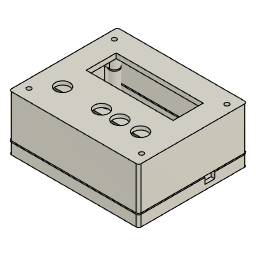
hotplate controller case v5 (Autodesk Fusion 360 design; units mm, degrees)
Autodesk Fusion 360 part; units mm, degrees
note: some values were not read from the file. Set by a fixed rule: which sketch regions a step uses.
sketch "Sketch1" plane through (0, 0, 0) normal (0, 0, 1) x (1, 0, 0)
  line L0 (0.5, 79.5) -> (106.9, 79.5)
  line L1 (106.9, 79.5) -> (106.9, -9.5)
  line L2 (106.9, -9.5) -> (0.5, -9.5)
  line L3 (0.5, -9.5) -> (0.5, 79.5)
  circle A0 centre (-121.3001, 1.3) radius 5
  line L4 (-51.3001, 1.3) -> (-121.3001, 1.3) construction
  line L5 (-139.5001, 79.5) -> (-33.1001, 79.5)
  circle A1 centre (-121.3001, 68.7) radius 1.8
  line L6 (-139.5001, -9.5) -> (-139.5001, 79.5)
  line L7 (-33.1001, 79.5) -> (-33.1001, -9.5)
  circle A2 centre (-51.3001, 1.3) radius 5
  line L8 (-51.3001, 68.7) -> (-51.3001, 1.3) construction
  line L9 (-121.3001, 1.3) -> (-121.3001, 68.7) construction
  circle A3 centre (-121.3001, 68.7) radius 5
  circle A4 centre (-51.3001, 1.3) radius 1.8
  circle A5 centre (-121.3001, 1.3) radius 1.8
  line L10 (-121.3001, 68.7) -> (-51.3001, 68.7) construction
  circle A6 centre (-51.3001, 68.7) radius 1.8
  line L11 (-136.5, 76.5) -> (-36.1001, 76.5)
  line L12 (-33.1001, -9.5) -> (-139.5001, -9.5)
  circle A7 centre (-51.3001, 68.7) radius 5
  circle A8 centre (-130, 62) radius 1.8
  circle A9 centre (-42, 62) radius 1.8
  circle A10 centre (-130, 8) radius 1.8
  circle A11 centre (-42, 8) radius 1.8
  circle A12 centre (-132.5001, 0) radius 1.8
  circle A13 centre (-132.5001, 70) radius 1.8
  circle A14 centre (-40.1001, 70) radius 1.8
  circle A15 centre (-40.1001, 0) radius 1.8
  line L13 (-136.5, 74) -> (-136.5, 76.5)
  line L14 (-132.5001, 74) -> (-136.5, 74)
  line L15 (-38.6001, 74) -> (-36.1001, 74)
  circle A16 centre (7.4999, 70) radius 1.8
  circle A17 centre (99.8999, 70) radius 1.8
  circle A18 centre (7.4999, 0) radius 1.8
  circle A19 centre (99.8999, 0) radius 1.8
  line L16 (-36.1001, 66) -> (-36.1001, 4)
  line L17 (-36.1001, -6.5) -> (-136.5001, -6.5)
  line L18 (-132.5001, 4) -> (-136.5, 4)
  line L19 (-134.0029, 66) -> (-136.5001, 66)
  line L20 (-36.1001, 76.5) -> (-36.1001, 74)
  line L21 (-40.0992, 66) -> (-36.1001, 66)
  line L22 (-38.6001, 4) -> (-36.1001, 4)
  line L23 (-36.1001, -4) -> (-40.0992, -4)
  line L24 (-36.1001, -4) -> (-36.1001, -6.5)
  line L25 (-134.0029, -4) -> (-136.5001, -4)
  line L26 (-136.5001, -4) -> (-136.5001, -6.5)
  line L27 (-136.5001, 66) -> (-136.5, 4)
  line L28 (-136.5, 15) -> (-139.5001, 15)
  line L29 (-136.5, 23) -> (-139.5001, 23)
  line L30 (-136.5, 45) -> (-139.5001, 45)
  line L31 (-136.5, 53) -> (-139.5001, 53)
  line L32 (7.4999, 4) -> (3.5, 4)
  arc A20 (7.4971, -4) -> (7.4999, 4) centre (7.4999, 0) ccw
  line L33 (7.4971, -4) -> (3.4999, -4)
  line L34 (3.4999, -4) -> (3.4999, -6.5)
  line L35 (103.8999, -6.5) -> (3.4999, -6.5)
  line L36 (103.8999, -4) -> (103.8999, -6.5)
  line L37 (103.8999, -4) -> (99.9008, -4)
  arc A21 (99.8999, 4) -> (99.9008, -4) centre (99.8999, 0) ccw
  line L38 (99.8999, 4) -> (103.8999, 4)
  line L39 (103.8999, 66) -> (103.8999, 4)
  line L40 (99.9008, 66) -> (103.8999, 66)
  arc A22 (99.8999, 74) -> (99.9008, 66) centre (99.8999, 70) ccw
  line L41 (99.8999, 74) -> (103.8999, 74)
  line L42 (103.8999, 76.5) -> (103.8999, 74)
  line L43 (3.5, 76.5) -> (103.8999, 76.5)
  line L44 (3.5, 74) -> (3.5, 76.5)
  line L45 (7.4999, 74) -> (3.5, 74)
  arc A23 (7.4971, 66) -> (7.4999, 74) centre (7.4999, 70) ccw
  line L46 (7.4971, 66) -> (3.4999, 66)
  line L47 (3.4999, 66) -> (3.5, 4)
  circle A24 centre (-132.5001, 0) radius 4
  circle A25 centre (-132.5001, 70) radius 4
  circle A26 centre (-40.1001, 0) radius 4
  circle A27 centre (-40.1001, 70) radius 4
  line L48 (-38.6001, 74) -> (-40.1001, 74)
  line L49 (-38.6001, 4) -> (-40.1001, 4)
  line L50 (-134.0029, -4) -> (-132.5001, -4)
  line L51 (-134.0029, 66) -> (-132.5001, 66)
  line L52 (3.5, 4) -> (3.4999, -4)
  line L53 (103.8999, 4) -> (103.8999, -4)
  line L54 (103.8999, 74) -> (103.8999, 66)
  line L55 (3.5, 74) -> (3.4999, 66)
  circle A28 centre (20, 15) radius 5.9
  circle A29 centre (52, 15) radius 5.9
  circle A30 centre (67, 15) radius 5.9
  circle A31 centre (84, 15) radius 5.9
  line L56 (17.9999, 61) -> (89.3999, 61)
  line L57 (89.3999, 61) -> (89.3999, 36.4)
  line L58 (89.3999, 36.4) -> (17.9999, 36.4)
  line L59 (17.9999, 36.4) -> (17.9999, 61)
  line L60 (89.3999, 60) -> (94.3999, 60)
  line L61 (94.3999, 60) -> (94.3999, 37.4)
  line L62 (94.3999, 37.4) -> (89.3999, 37.4)
  line L63 (14, 67) -> (94.3999, 67)
  line L64 (94.3999, 67) -> (94.3999, 31.9055)
  line L65 (94.3999, 31.9055) -> (14, 31.9055)
  line L66 (14, 31.9055) -> (14, 67)
  circle A32 centre (8, 15) radius 1.8
  circle A33 centre (37, 15) radius 1.8
  circle A34 centre (96, 15) radius 1.8
  circle A35 centre (37, 15) radius 4
  line L67 (-33.1001, 53) -> (-36.1001, 53)
  line L68 (-33.1001, 45) -> (-36.1001, 45)
  circle A36 centre (8, 15) radius 4
  circle A37 centre (8, 15) radius 1.8
  circle A38 centre (37, 15) radius 1.8
  circle A39 centre (37, 15) radius 4
  circle A40 centre (96, 15) radius 4
  circle A41 centre (96, 15) radius 1.8
  circle A42 centre (157, 15) radius 1.8
  circle A43 centre (128, 15) radius 1.8
  line L69 (124, 22) -> (124, 8)
  circle A44 centre (187, 15) radius 1
  circle A45 centre (140, 15) radius 1
  circle A46 centre (172, 15) radius 1
  circle A47 centre (157, 15) radius 1.8
  circle A48 centre (216, 15) radius 1.8
  circle A49 centre (204, 15) radius 1
  circle A50 centre (216, 15) radius 1.8
  circle A51 centre (128, 15) radius 1.8
  line L70 (124, 22) -> (220, 22)
  line L71 (220, 22) -> (220, 8)
  line L72 (220, 8) -> (124, 8)
  circle A52 centre (137.9, 11.5) radius 0.75
  circle A53 centre (142.1, 11.5) radius 0.75
  circle A54 centre (174.1, 11.5) radius 0.75
  circle A55 centre (169.9, 11.5) radius 0.75
  circle A56 centre (189.1, 11.5) radius 0.75
  circle A57 centre (184.9, 11.5) radius 0.75
  circle A58 centre (206.1, 11.5) radius 0.75
  circle A59 centre (201.9, 11.5) radius 0.75
  point P0 (-120, 0)
  dimension "d22" = 3.6
  dimension "d23" = 3.6
  dimension "d24" = 3.6
  dimension "d25" = 3.6
  dimension "d30" = 10
  dimension "d31" = 10
  dimension "d32" = 10
  dimension "d43" = 3.6
  dimension "d44" = 3.6
  dimension "d59" = 11.8
  dimension "d60" = 11.8
  dimension "d61" = 11.8
  dimension "d62" = 11.8
  dimension "d68" = 71.4
  dimension "d69" = 5
  dimension "d70" = 24.6
  dimension "d97" = 2
  dimension "d98" = 2
  dimension "d99" = 2
  dimension "d100" = 2
  constraint coincident L8.start L10.end
  constraint coincident L4.start A2.centre
  constraint coincident A1.centre L9.end
  constraint coincident A0.centre L4.end
  constraint concentric A1 A3
  constraint concentric A0 A5
  constraint concentric A2 A4
  constraint concentric A6 A7
  constraint perpendicular L15 L20
  constraint perpendicular L16 L21
  constraint perpendicular L17 L24
  constraint perpendicular L17 L26
  constraint coincident L6 L28.end
  constraint perpendicular L6 L28
  constraint coincident L6 L29.end
  constraint perpendicular L6 L29
  constraint coincident L27 L29.start
  constraint coincident L27 L28.start
  constraint coincident L6 L30.end
  constraint perpendicular L6 L30
  constraint coincident L6 L31.end
  constraint perpendicular L6 L31
  constraint coincident L27 L31.start
  constraint coincident L27 L30.start
  constraint tangent L45 A23
  constraint perpendicular L41 L42
  constraint perpendicular L39 L40
  constraint tangent A21 L38
  constraint perpendicular L35 L36
  constraint perpendicular L34 L35
  constraint coincident L18.start A24
  constraint tangent L18 A24
  constraint concentric A13 A25
  constraint coincident L14.start A25
  constraint tangent L14 A25
  constraint concentric A15 A26
  constraint coincident L23.end A26
  constraint concentric A14 A27
  constraint coincident L21.start A27
  constraint coincident A27 L48.end
  constraint tangent A27 L48
  constraint parallel L15 L48
  constraint coincident A26 L49.end
  constraint tangent A26 L49
  constraint horizontal L49
  constraint coincident A24 L50.end
  constraint tangent A24 L50
  constraint coincident A25 L51.end
  constraint tangent A25 L51
  constraint perpendicular L37 L53
  constraint perpendicular L40 L54
  constraint horizontal L56
  constraint vertical L57
  constraint horizontal L58
  constraint vertical L59
  constraint horizontal L60
  constraint vertical L61
  constraint horizontal L62
  constraint coincident L57 L60.start
  constraint coincident L57 L62.end
  constraint horizontal L63
  constraint vertical L64
  constraint horizontal L65
  constraint vertical L66
  constraint concentric A33 A35
  constraint coincident L7 L67.start
  constraint perpendicular L7 L67
  constraint coincident L7 L68.start
  constraint coincident L16 L67.end
  constraint coincident L16 L68.end
  constraint concentric A36 A37
  constraint concentric A40 A41
  constraint concentric A38 A39
  constraint horizontal L70
  constraint vertical L71
  constraint horizontal L72
  measures "d22" diameter of A6
  measures "d23" diameter of A4
  measures "d24" diameter of A1
  measures "d25" diameter of A5
  measures "d30" diameter of A0
  measures "d31" diameter of A2
  measures "d32" diameter of A7
  measures "d43" diameter of A12
  measures "d44" diameter of A13
  measures "d59" diameter of A28
  measures "d60" diameter of A29
  measures "d61" diameter of A30
  measures "d62" diameter of A31
  measures "d68" distance of L56.start L56.end
  measures "d69" distance of L61.end L62.end
  measures "d70" distance of L56.start L58.end
  measures "d97" diameter of A45
  measures "d98" diameter of A46
  measures "d99" diameter of A44
  measures "d100" diameter of A49
extrude "Extrude1" add sketch "Sketch1" along normal blind 3 contours L11 L13 L14 L15 L16 L17 L18 L19 L20 L21 L22 L23 L24 L25 L26 L27 A24 A25 A26 A27 L48 L49 L50 L51 makes body 1
extrude "Extrude2" add sketch "Sketch1" along normal blind 9 contours L5 L6 L7 L11 L13 L14 L15 L16 L19 L20 L21 L27 L31 A25 A27 L48 L51 L67 | L6 L27 L29 L30 | L6 L7 L12 L16 L17 L18 L22 L23 L24 L25 L26 L27 L28 A24 A26 L49 L50 L68 bodies 1
extrude "Extrude3" add sketch "Sketch1" along normal blind 4 contours L5 L6 L7 L11 L13 L14 L15 L16 L19 L20 L21 L27 L31 A25 A27 L48 L51 L67 | L6 L27 L30 L31 | L7 L16 L67 L68 | L6 L27 L28 L29 bodies 1
extrude "Extrude4" add sketch "Sketch1" along normal blind 7 contours A0 | A2 | A3 | A7 bodies 1
extrude "Extrude6" add sketch "Sketch1" along normal blind 25 contours A27 | A25 | A26 | A24 bodies 1
chamfer "Chamfer1" distance 1.5 angle 45 4 edges at (-131.6782, 62.6509, 3) (-43.6782, 62.6509, 3) (-43.6782, 8.6509, 3) (-131.6782, 8.6509, 3) on bodies 1
extrude "Extrude5" add sketch "Sketch1" against normal blind 35 separate body contours L0 L1 L2 L3 makes body 2
extrude "Extrude7" add sketch "Sketch1" against normal blind 3 contours L32 A20 L33 L34 L35 L36 L37 A21 L38 L39 L40 A22 L41 L42 L43 L44 L45 A23 L46 L47 bodies 2
extrude "Extrude8" add sketch "Sketch1" against normal blind 4 contours L56 L57 L58 L59 L60 L62 L63 L64 L65 L66 bodies 2
extrude "Extrude9" add sketch "Sketch1" against normal blind 1 contours L57 L60 L61 L62 L64 bodies 2
extrude "Extrude10" add sketch "Sketch1" against normal blind 9 contours A35 A39 | A36 | A40 bodies 2
extrude "Extrude11" add sketch "Sketch1" against normal blind 2 contours A32 A37 | A33 A38 | A34 A41 bodies 2
extrude "Extrude12" add sketch "Sketch1" against normal blind 19 contours L32 A20 L33 L52 | L45 A23 L46 L55 | L37 A21 L38 L53 | L40 A22 L41 L54 bodies 2
fillet "Fillet1" radius 2 8 edges at (-33.1001, -9.5, 4.5) (-33.1001, 79.5, 4.5) (-139.5001, -9.5, 4.5) (-139.5001, 79.5, 4.5) (0.5, -9.5, -17.5) (0.5, 79.5, -17.5) (106.9, -9.5, -17.5) (106.9, 79.5, -17.5) on bodies 1 2
move_body "Move1" bodies 2 to x (1, 0, 0) y (0, 1, 0) z (0, 0, 1) at (-140, 0, 45)
extrude "Extrude13" add sketch "Sketch1" along normal blind 3 separate body contours L69 L70 L71 L72 makes body 3
fillet "Fillet2" radius 4 4 edges at (220, 8, 1.5) (220, 22, 1.5) (124, 8, 1.5) (124, 22, 1.5) on bodies 3
move_body "Move2" bodies 3 to x (1, 0, 0) y (0, 1, 0) z (0, 0, 1) at (-260, 0, 31)
equation "d36 = 3 mm + 3 mm + 3 mm"
equation "d89 = -30 mm + 11 mm"
